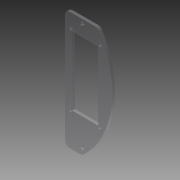
# Autodesk Inventor part: LCD Plate
Saved by Autodesk Inventor 2015 (Build 190159000, 159)
## iProperties
Created: 2016-02-21
Part Number: LCD Plate
Material: Polycarbonate, Clear
Document SubType Name: Modeling
Designer: James Yelland
Density: 1.2 g/cm^3
Appearance: Polycarbonate - Clear
Author: James Yelland
Autodesk Inventor part; units mm, degrees
ref_plane "YZ Plane" through (0, 0, 0) normal (1, 0, 0) x (0, 1, 0)
ref_plane "XZ Plane" through (0, 0, 0) normal (0, 1, 0) x (-1, 0, 0)
ref_plane "XY Plane" through (0, 0, 0) normal (0, 0, 1) x (1, 0, 0)
sketch "Sketch1" plane through (0, 0, 0) normal (0, 1, 0) x (-1, 0, 0)
  circle A0 centre (-34.3765, 114.6665) radius 1.6
  circle A1 centre (-34.8464, 1.7591) radius 1.6
  arc A2 (-53.1019, 117.2341) -> (-38.3819, -1.7764) centre (30.561, 67.1665) ccw
  line L0 (-34.3765, 119.6665) -> (-48.8115, 119.6665)
  arc A3 (-38.3819, -1.7764) -> (-36.4764, -3.6306) centre (30.561, 67.1665) ccw
  line L1 (-33.0386, -5) -> (-21.9122, -5)
  line L2 (-16.9122, 0.0037) -> (-16.9963, 114.6702)
  line L3 (-21.9963, 119.6665) -> (-34.3765, 119.6665)
  arc A4 (-48.8115, 119.6665) -> (-53.1019, 117.2341) centre (-48.8115, 114.6665) ccw
  arc A5 (-36.4764, -3.6306) -> (-33.0386, -5) centre (-33.0386, 0) ccw
  circle A6 centre (-22.239, 104.2134) radius 1.25
  circle A7 centre (-53.239, 104.2134) radius 1.25
  circle A8 centre (-53.239, 29.2134) radius 1.25
  circle A9 centre (-22.239, 29.2134) radius 1.25
  line L4 (-24.639, 102.8634) -> (-24.639, 30.5634)
  line L5 (-24.639, 30.5634) -> (-51.939, 30.5634)
  line L6 (-51.939, 30.5634) -> (-51.939, 102.8634)
  line L7 (-51.939, 102.8634) -> (-24.639, 102.8634)
  arc A10 (-21.9122, -5) -> (-16.9122, 0.0037) centre (-21.9122, 0) ccw
  arc A11 (-16.9963, 114.6702) -> (-21.9963, 119.6665) centre (-21.9963, 114.6665) ccw
  point P0 (0, 0)
  constraints: 16 end point, 12 centre point, 12 point on circle
extrude "Extrusion1" add sketch "Sketch1" along normal blind 3
body "Solid1"
